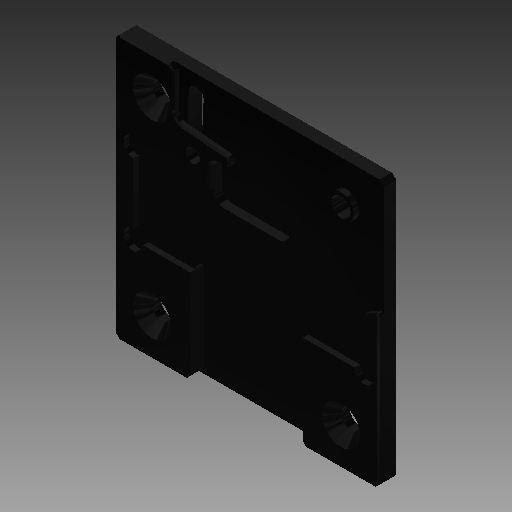
# Autodesk Inventor part: JF-GM-VL-0041
Saved by Autodesk Inventor 2018.3 (Build 223284000, 284)
## iProperties
Created: 2010-11-11
Part Number: JF-GM-VL-0041
Document SubType Name: Modeling
Designer: COOPB
Density: 2.71 g/cm^3
Material: ALUMINUM, 6061-T6
Mass: 110.455 g
Surface Area: 187.659 cm^2
Volume: 40.7583 cm^3
Checked By: COOPB
Engr Approved By: COOPB
Description: SLIDE MOUNTING PLATE
Vendor: HHMI JFRC
Engineer: COOPB
Appearance: Glossy - Black
Author: COOPB
Revision Number: 0
Autodesk Inventor part; units mm, degrees
note: some values were not read from the file. Chosen so that the rebuilt part matches the saved one: sketch regions of "Extrusion2".
ref_plane "YZ Plane" through (0, 0, 0) normal (1, 0, 0) x (0, 1, 0)
ref_plane "XZ Plane" through (0, 0, 0) normal (0, 1, 0) x (-1, 0, 0)
sketch "Sketch1" plane through (0, 0, 0) normal (0, 0, 1) x (1, 0, 0)
  line L0 (0, 62.23) -> (0, -62.23) construction
  line L1 (-63.4058, 0) -> (69.2849, 0) construction
  line L2 (-44.45, 44.45) -> (44.45, 44.45)
  line L3 (44.45, 44.45) -> (44.45, -44.45)
  line L4 (44.45, -44.45) -> (-44.45, -44.45)
  line L5 (-44.45, -44.45) -> (-44.45, 44.45)
  line L6 (31.75, 31.75) -> (-31.75, 31.75) construction
  line L7 (-31.75, 31.75) -> (-31.75, -31.75) construction
  line L8 (-31.75, -31.75) -> (31.75, -31.75) construction
  line L9 (31.75, -31.75) -> (31.75, 31.75) construction
  line L10 (-38.1, 14.224) -> (39.624, 14.224)
  line L11 (39.624, 14.224) -> (39.624, -12.7)
  line L12 (39.624, -12.7) -> (-38.1, -12.7)
  line L13 (-38.1, -12.7) -> (-38.1, 14.224)
  circle A0 centre (-38.1, 14.224) radius 3.302
  circle A1 centre (-38.1, -12.7) radius 3.302
  line L14 (-19.05, -13.208) -> (-19.05, -44.45)
  line L15 (-19.05, -44.45) -> (19.05, -44.45)
  line L16 (19.05, -44.45) -> (19.05, -13.208)
  line L17 (-12.7, 13.208) -> (-12.7, 20.574)
  arc A2 (-9.398, 23.876) -> (-12.7, 20.574) centre (-9.398, 20.574) ccw
  line L18 (-9.398, 23.876) -> (9.398, 23.876)
  arc A3 (12.7, 20.574) -> (9.398, 23.876) centre (9.398, 20.574) ccw
  line L19 (12.7, 20.574) -> (12.7, 13.208)
  line L20 (-9.398, 9.906) -> (9.398, 9.906)
  line L21 (-15.748, -9.906) -> (15.748, -9.906)
  arc A4 (-12.7, 13.208) -> (-9.398, 9.906) centre (-9.398, 13.208) ccw
  arc A5 (9.398, 9.906) -> (12.7, 13.208) centre (9.398, 13.208) ccw
  arc A6 (-15.748, -9.906) -> (-19.05, -13.208) centre (-15.748, -13.208) ccw
  arc A7 (19.05, -13.208) -> (15.748, -9.906) centre (15.748, -13.208) ccw
  line L22 (-38.1, -12.7) -> (38.1, -12.7)
  line L23 (38.1, -12.7) -> (38.1, 12.7)
  line L24 (38.1, 12.7) -> (-38.1, 12.7)
  line L25 (-38.1, 12.7) -> (-38.1, -12.7)
  line L26 (-38.1, -12.7) -> (38.1, 12.7) construction
  arc A8 (38.1, 12.7) -> (49.4215, 22.2135) centre (31.75, 31.75) ccw construction
  arc A9 (40.8788, 8.0472) -> (47.7671, 12.0368) centre (31.75, 31.75) ccw
  line L27 (47.7671, 12.0368) -> (38.8331, 34.5596)
  line L28 (28.7639, 18.6118) -> (26.4225, 24.5144)
  circle A10 centre (31.75, 31.75) radius 4.3656
  line L29 (31.75, 31.75) -> (35.9321, 21.2069) construction
  arc A11 (38.8331, 34.5596) -> (31.6627, 39.3695) centre (31.75, 31.75) ccw
  line L30 (31.6627, 39.3695) -> (-18.9391, 38.7898)
  arc A12 (-18.9391, 38.7898) -> (-19.4465, 32.487) centre (-18.9028, 35.6151) ccw
  line L31 (-19.4465, 32.487) -> (26.4225, 24.5144)
  line L32 (-18.9028, 35.6151) -> (31.75, 31.75) construction
  line L33 (31.75, 31.75) -> (26.4225, 24.5144) construction
  circle A13 centre (39.624, -12.7) radius 3.302
  line L34 (-7.1755, 27.1717) -> (-24.638, 28.6995)
  circle A14 centre (31.75, 31.75) radius 4.3148
  arc A15 (40.8788, 8.0472) -> (28.7639, 18.6118) centre (1.8543, -24.4755) ccw
  line L35 (39.624, 4.327) -> (44.45, 7.1133)
  line L36 (-24.638, 28.6995) -> (-24.638, 44.45)
  arc A16 (-16.1868, 37.8508) -> (-15.9605, 24.0774) centre (31.75, 31.75) ccw
  arc A17 (-21.1002, 38.4762) -> (-20.8507, 23.291) centre (31.75, 31.75) ccw
  arc A18 (-20.8507, 23.291) -> (-15.9605, 24.0774) centre (-18.4056, 23.6842) ccw
  arc A19 (-18.9028, 35.6151) -> (-18.4056, 23.6842) centre (31.75, 31.75) ccw construction
  circle A20 centre (-18.9028, 35.6151) radius 2.3813
  line L37 (-19.006, 29.635) -> (-19.2777, 36.1557) construction
  circle A21 centre (-18.0554, 21.7467) radius 2.3749 construction
  line L38 (-18.0554, 21.7467) -> (-18.0912, 21.7395) construction
  arc A22 (-16.1868, 37.8508) -> (-21.1002, 38.4762) centre (-18.6435, 38.1635) ccw
  arc A23 (-7.3194, 23.876) -> (-7.1755, 27.1717) centre (-7.3194, 25.527) ccw
  line L39 (-7.3194, 23.876) -> (-7.3194, 4.327)
  line L40 (-7.3194, 4.327) -> (39.624, 4.327)
  line L41 (-38.1, 12.3) -> (36.9, 12.3)
  line L42 (36.9, 12.3) -> (36.9, -12.7)
  point P0 (0, 31.75)
  point P1 (0, -31.75)
  point P2 (-31.75, 0)
  point P3 (31.75, 0)
  dimension "d0" = 88.9
  dimension "d1" = 63.5
  dimension "d2" = 6.604
  dimension "d6" = 25.4
  dimension "d8" = 19.812
  dimension "d11" = 25.4
  dimension "d12" = 76.2
  dimension "d13" = 1.524
  dimension "d14" = 1.524
  dimension "d15" = 25.4
  dimension "d17" = 15.24
  dimension "d18" = 3.175
  dimension "d23" = 23.876
  dimension "d36" = 50.8
  dimension "d37" = 116
  dimension "d38" = 8.7312
  dimension "d55" = 116.503
  dimension "d58" = 5
  dimension "d59" = 0.0508
  dimension "d60" = 6.35
  dimension "d61" = 50.8
  dimension "d62" = 7.874
  dimension "d63" = 4.86
  dimension "d67" = 2.286
  dimension "d68" = 120
  dimension "d69" = 19.812
  dimension "d71" = 4.953
  dimension "d73" = 4.7625
  dimension "d77" = 38.1
  dimension "d78" = 4.7498
  dimension "d87" = 0.508
  dimension "d88" = 3.81
  dimension "d89" = 1.651
  dimension "d93" = 22.7033
  dimension "d94" = 25
  dimension "d95" = 75
  dimension "d96" = 38.7816
  constraints: 83 end point, 37 point on circle, 24 centre point, 23 tangent, 18 coincident, 15 parallel, 13 perpendicular, 8 equal radius, 7 point on line, 4 midpoint, 3 horizontal, 12 other
  measures "d0" distance between parallel lines of L4 L2
  measures "d1" distance between parallel lines of L8 L6
  measures "d2" diameter of A0
  measures "d6" distance between parallel lines of L19 L17
  measures "d8" distance between parallel lines of L21 L20
  measures "d11" distance between parallel lines of L22 L24
  measures "d12" distance between parallel lines of L23 L25
  measures "d13" distance between parallel lines of L10 L24
  measures "d14" distance between parallel lines of L11 L23
  measures "d15" radius of A9
  measures "d17" distance between parallel lines of L28 L27
  measures "d18" radius of A12
  measures "d23" distance between parallel lines of L1 L18
  measures "d36" distance of L32.start L32.end
  measures "d37" angle of L32 L29
  measures "d38" diameter of A10
  measures "d55" angle of L33 L31
  measures "d58" angle of L18 L34
  measures "d59" radial gap between concentric circles of A10 A14
  measures "d60" distance of L28.start L28.end
  measures "d61" radius of A15
  measures "d62" distance from line of A9.start L27
  measures "d63" angle of L34 L31
  measures "d67" distance edge to line of A9 L35
  measures "d68" angle of L11 L35
  measures "d69" distance between parallel lines of L5 L36
  measures "d71" radial gap between concentric circles of A17 A16
  measures "d73" diameter of A20
  measures "d77" distance between parallel lines of L16 L14
  measures "d78" diameter of A21
  measures "d87" distance edge to line of A18 L38
  measures "d88" distance edge to line of A22 L2
  measures "d89" radius of A23
  measures "d93" distance from line of L38.start L2
  measures "d94" distance between parallel lines of L22 L41
  measures "d95" distance between parallel lines of L13 L42
extrude "Extrusion1" add sketch "Sketch1" against normal blind 6.35 contours L2 L36 L34 A17 A18 A16 A23 L18 A2 L17 L10 A0 L13 A1 L12 A6 L14 L4 L5 | L2 L3 L27 A11 L30 A22 A17 A12 L34 L36 | L14 A6 L12 A7 L16 L4 | L3 A9 A15 L11 L10 L28 L31 A16 A22 L30 A11 L27 | A17 A12 L31 A16 L34 | L34 A16 A18 A17 | L16 A7 L12 A13 L11 L35 L3 L4 | L3 L35 L11 A15 A9 | A16 L31 L28 A15 L10 L19 A3 L18 A23 L34 | A17 A12 L30 A22 A16 L31 | A12 A17 | A6 L21 A7 L12 | L12 A1 L13 A0 L41 A4 L20 L39 L40 L42 A13 A7 L21 A6 | A17 A22 L30 A12 | A1 L13 L12 | L12 L13 A1 | L40 L23 A15 L11 | L11 A13 L23 L40 | A15 L23 L24 L10 L11 | L39 L10 L17 A2 L18 | L18 A3 L19 L10 L39 | A13 L42 L12 | L12 L11 A13 | L11 L12 L23 A13 | L40 L42 A15 L23 | L23 A13 L42 L40 | A15 L24 L23 | L39 L24 A4 L17 L10 | L10 L19 A5 L24 L39 | L42 A13 L23 L12 | A0 L10 L13 | L13 L41 A0 | L40 L39 L20 A5 L41 L42 | A15 L24 A5 L19 L10 | L41 A5 L24 A15 | L17 A4 L24 A0 L10 | L39 L41 A4 L24 | L24 A5 L41 L39 | L13 L24 A0 L41 | A0 L24 L13 L10 | A0 L24 A4 L41 | A5 L20 L39 L41 | L39 L20 A4 L41 | A10 | A14 | A20
extrude "Extrusion2" cut sketch "Sketch1" against normal blind 1.778 contours L2 L3 L27 A11 L30 A22 A17 A12 L34 L36 | L14 A6 L12 A7 L16 L4 | L3 A9 A15 L11 L10 L28 L31 A16 A22 L30 A11 L27 | A17 A12 L31 A16 L34 | L3 L35 L11 A15 A9 | A16 L31 L28 A15 L10 L19 A3 L18 A23 L34 | A17 A12 L30 A22 A16 L31 | A12 A17 | A6 L21 A7 L12 | L12 A1 L13 A0 L41 A4 L20 L39 L40 L42 A13 A7 L21 A6 | A17 A22 L30 A12 | A1 L13 L12 | L12 L13 A1 | L40 L23 A15 L11 | L11 A13 L23 L40 | A15 L23 L24 L10 L11 | L39 L10 L17 A2 L18 | L18 A3 L19 L10 L39 | A13 L42 L12 | L12 L11 A13 | L11 L12 L23 A13 | L40 L42 A15 L23 | L23 A13 L42 L40 | A15 L24 L23 | L39 L24 A4 L17 L10 | L10 L19 A5 L24 L39 | L42 A13 L23 L12 | A0 L10 L13 | L13 L41 A0 | L40 L39 L20 A5 L41 L42 | A15 L24 A5 L19 L10 | L41 A5 L24 A15 | L17 A4 L24 A0 L10 | L39 L41 A4 L24 | L24 A5 L41 L39 | L13 L24 A0 L41 | A0 L24 L13 L10 | A0 L24 A4 L41 | A5 L20 L39 L41 | L39 L20 A4 L41 | A10 | A20
extrude "Extrusion3" cut sketch "Sketch1" against normal blind 4.572 contours L14 A6 L12 A7 L16 L4 | A6 L21 A7 L12 | L39 L10 L17 A2 L18 | L18 A3 L19 L10 L39 | L39 L24 A4 L17 L10 | L10 L19 A5 L24 L39 | L39 L41 A4 L24 | L24 A5 L41 L39 | A5 L20 L39 L41 | L39 L20 A4 L41
extrude "Extrusion4" cut sketch "Sketch1" against normal up to surface (4.572 mm away) from surface at -1.778 contours A17 A12 L31 A16 L34 | L34 A16 A18 A17 | A17 A12 L30 A22 A16 L31 | A17 A22 L30 A12 | A20
fillet "Fillet1" radius 3.302 1 edges at (-24.638, 28.6995, -0.889)
fillet "Fillet2" radius 0.762 2 edges at (-7.1755, 27.1717, -0.889) (44.45, 7.1133, -0.889)
hole "Hole1" at (-31.75, 31.75, 0) at (-31.75, -31.75, 0) at (31.75, -31.75, 0) direction (0, 0, -1) diameter 6.7564 depth 25.4 tip angle 118 countersink diameter 12.8778 countersink angle 82 clearance for "Flat Head Machine Screw (82)" size "1/4" standard "Ansi Unified Screw Threads"
hole "Hole2" at (31.75, 31.75, 0) direction (0, 0, -1) diameter 6.5278 end through all clearance for "Hex Head Bolt" size "1/4" standard "Ansi Unified Screw Threads"
hole "Hole3" at (-18.0554, 21.7467, 0) direction (0, 0, -1) diameter 4.7498 end through all
chamfer "Chamfer1" distance 1.524 angle 45 7 edges at (-44.45, -44.45, -3.175) (-44.45, 44.45, -3.175) (44.45, 44.45, -4.064) (44.45, -44.45, -3.175) (-19.05, -44.45, -2.286) (19.05, -44.45, -2.286) (-24.638, 44.45, -0.889)
ref_plane "Work Plane1" through (-19.006, 29.635, 0) normal (0.9991329, 0.0416345, 0) x (-0.0416345, 0.9991329, 0)
ref_plane "Work Plane2" through (0, 0, -4.064) normal (0, 0, 1) x (1, 0, 0)
chamfer "Chamfer2" distance 0.508 angle 45 29 edges at (-19.05, -28.067, 0) (-19.0402, -12.9532, 0) (-19.812, -43.688, 0) (-31.75, -44.45, 0) (-43.688, -43.688, 0) (-44.45, 0, 0) (-43.688, 43.688, 0) (-34.544, 44.45, 0) (-25.4, 43.688, 0) (-24.638, 37.3256, 0) (-23.7705, 29.4944, 0) (-14.3997, 27.8037, 0) (-5.67, 25.455, 0) (-8.3587, 23.876, 0) (-11.7329, 22.9089, 0) (-12.7, 17.399, 0) (31.75, -44.45, 0) (43.688, -43.688, 0) (44.45, -18.5663, 0) (44.069, 6.4534, 0) (41.4655, 5.3902, 0) (44.45, 0, -6.35) (43.688, 43.688, -6.35) (0, 44.45, -6.35) (-43.688, 43.688, -6.35) (-44.45, 0, -6.35) (-43.688, -43.688, -6.35) (0, -44.45, -6.35) (43.688, -43.688, -6.35)
body "Solid1"
